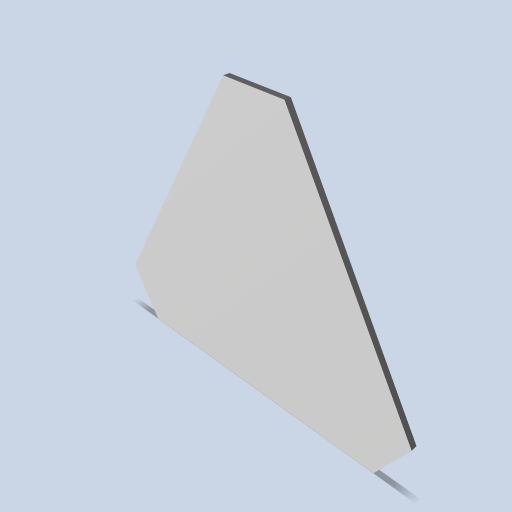
# Autodesk Inventor part: Triangle Base
Saved by Autodesk Inventor 2023 (Build 270158000, 158)
## iProperties
Created: 2022-10-16
Part Number: Triangle Base
Material: Generic
Document SubType Name: Modeling
Designer: Nathan
Density: 1 g/cm^3
Appearance: Smooth - White
Author: Nathan
Autodesk Inventor part; units mm, degrees
ref_plane "YZ Plane" through (0, 0, 0) normal (1, 0, 0) x (0, 1, 0)
ref_plane "XZ Plane" through (0, 0, 0) normal (0, 1, 0) x (-1, 0, 0)
ref_plane "XY Plane" through (0, 0, 0) normal (0, 0, 1) x (1, 0, 0)
sketch "Sketch1" plane through (0, 0, 0) normal (0, 0, 1) x (1, 0, 0)
  circle A0 centre (0, 0) radius 332.74
  line L0 (0, 665.48) -> (-576.3226, -332.74)
  line L1 (-576.3226, -332.74) -> (576.3226, -332.74)
  line L2 (576.3226, -332.74) -> (0, 665.48)
  line L3 (-488.3344, -180.34) -> (-400.3462, -332.74)
  line L4 (-444.3403, -256.54) -> (-576.3226, -332.74)
  line L5 (400.3462, -332.74) -> (488.3344, -180.34)
  line L6 (-87.9882, 513.08) -> (87.9882, 513.08)
  point P0 (444.3403, -256.54)
  point P1 (0, 513.08)
  dimension "d0" = 665.48
  dimension "d1" = 60
  dimension "d2" = 60
  dimension "d3" = 60
  dimension "d4" = 60
  dimension "d5" = 152.4
  dimension "d6" = 60
  dimension "d7" = 152.4
  dimension "d8" = 152.4
  constraints: 14 end point, 6 point on line, 3 midpoint, 3 tangent, 2 horizontal, 1 centre point, 1 coincident
  measures "d0" diameter of A0
  measures "d1" angle of L1 L0
  measures "d2" angle of L1 L2
  measures "d3" angle of L2 L0
  measures "d4" angle of L1 L3
  measures "d5" distance of L4.start L0.end
  measures "d6" angle of L1 L5
  measures "d7" distance of point (444.34, -256.54) L1.end
  measures "d8" distance of point (0, 513.08) L0.start
extrude "Extrusion1" add sketch "Sketch1" along normal blind 18.0086 contours A0 | A0 L2 L5 L1 | A0 L0 L6 L2 | L1 L3 L0 A0
body "Solid1"
